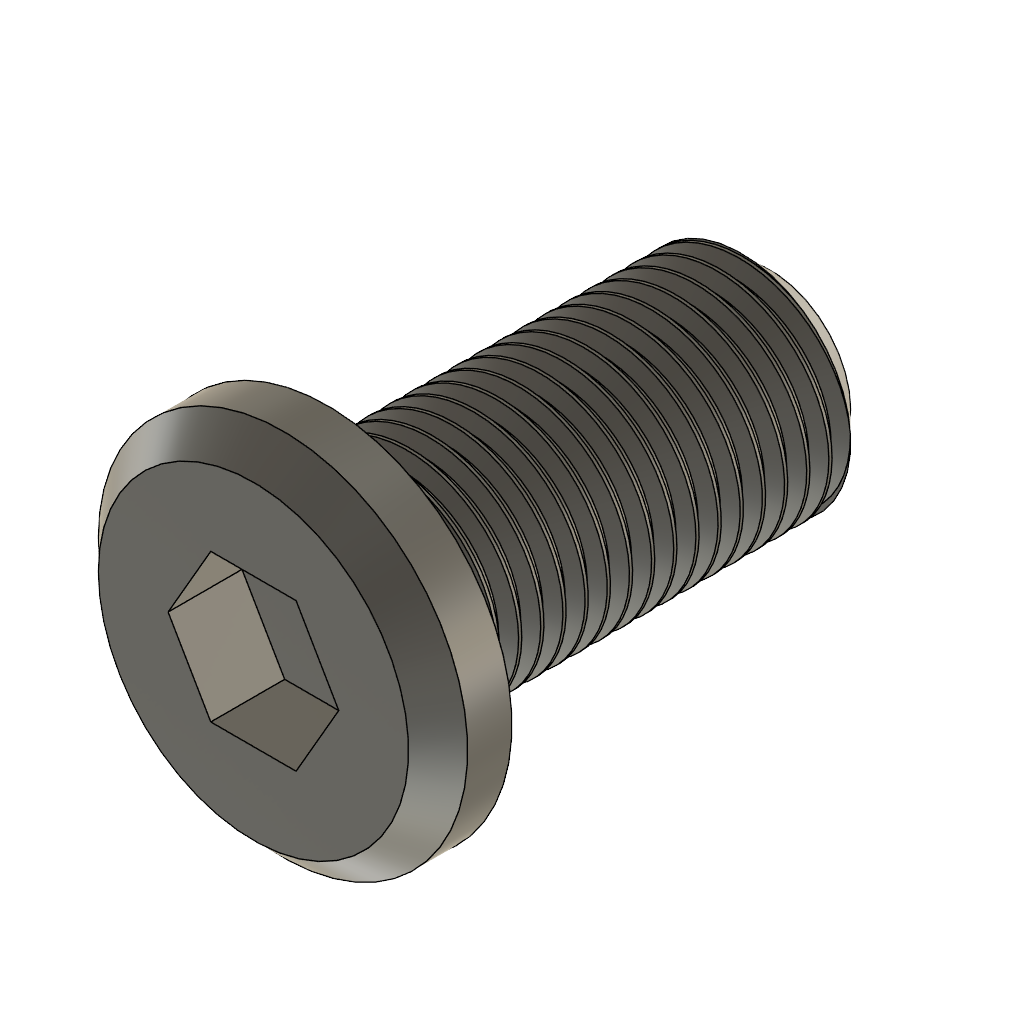
Threaded Bolts (Autodesk Fusion 360 design; units mm, degrees)
part number: 2026-01-26-22-27-08-883
Autodesk Fusion 360 part; units mm, degrees
sketch "Sketch8" plane through (0, 0, 0) normal (0, 1, 0) x (1, 0, 0)
  circle A0 centre (0, 0) radius 7.5
  dimension "d18" = 15
  constraint coincident A0.centre origin
  measures "d18" diameter of A0
extrude "Extrude5" add sketch "Sketch8" along normal blind 30
sketch "Sketch9" plane through (0, 0, 0) normal (0, -1, 0) x (1, 0, 0)
  circle A0 centre (0, 0) radius 7.5
  circle A1 centre (0, 0) radius 12.5
  dimension "d21" = 25
  constraint concentric A0 A1
  measures "d21" diameter of A1
extrude "Extrude6" add sketch "Sketch9" along normal blind 5 contours A0 | A1
chamfer "Chamfer2" distance 2 angle 45 2 edges at (-11.6541, -5, -4.5202) (-6.9925, 30, 2.7121) tangent chain off
thread "Thread2" "ISO Metric profile 15.0 M15x1.5 M15x1.5 6g" major diameter 14.85 minor diameter 13.1369 pitch 1.5 angle 60 modelled right hand crest width 0.2152 on face at (7.4907, 18.6667, 0.3738) crest through (7.425, -0.375, 0)
sketch "Sketch10" plane through (0, -5, 0) normal (0, -1, 0) x (1, 0, 0)
  circle A0 centre (0, 0) radius 10.5
  line L0 (-2.8868, 5) -> (-5.7735, 0)
  line L1 (-5.7735, 0) -> (-2.8868, -5)
  line L2 (-2.8868, -5) -> (2.8868, -5)
  line L3 (2.8868, -5) -> (5.7735, 0)
  line L4 (5.7735, 0) -> (2.8868, 5)
  line L5 (2.8868, 5) -> (-2.8868, 5)
  dimension "d27" = 5
  constraint coincident A0.centre origin
  measures "d27" distance of A0.centre L5
extrude "Extrude7" cut sketch "Sketch10" against normal blind 5 contours L0 L1 L2 L3 L4 L5
